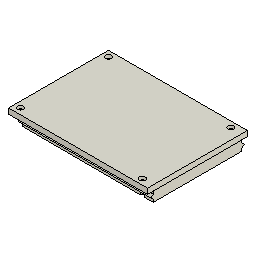
Crashsense Mark-1 LID v10 (Autodesk Fusion 360 design; units mm, degrees)
Autodesk Fusion 360 part; units mm, degrees
note: some values were not read from the file. Chosen so that the rebuilt part matches the saved one: which bodies a step acts on; which face or edge a step refers to. Set by a fixed rule: which sketch regions a step uses.
sketch "Sketch1" plane through (0, 0, 0) normal (0, 0, 1) x (1, 0, 0)
  line L0 (64.0125, -46.025) -> (-64.0125, -46.025)
  line L1 (-64.0125, -46.025) -> (-64.0125, 46.025)
  line L2 (-64.0125, 46.025) -> (64.0125, 46.025)
  line L3 (64.0125, 46.025) -> (64.0125, -46.025)
  line L4 (64.0125, -46.025) -> (-64.0125, 46.025) construction
  line L5 (-64.0125, -46.025) -> (64.0125, 46.025) construction
  line L6 (54.0125, -36.025) -> (-54.0125, -36.025)
  line L7 (-54.0125, -36.025) -> (-54.0125, 36.025)
  line L8 (-54.0125, 36.025) -> (54.0125, 36.025)
  line L9 (54.0125, 36.025) -> (54.0125, -36.025)
  line L10 (54.0125, -36.025) -> (-54.0125, 36.025) construction
  line L11 (-54.0125, -36.025) -> (54.0125, 36.025) construction
  line L12 (54.0125, -36.025) -> (64.0125, -36.025)
  line L13 (54.0125, -36.025) -> (54.0125, -46.025)
  line L14 (54.0125, -46.025) -> (64.0125, -46.025)
  line L15 (54.0125, 36.025) -> (54.0125, 46.025)
  line L16 (54.0125, 36.025) -> (64.0125, 36.025)
  line L17 (-54.0125, 36.025) -> (-64.0125, 36.025)
  line L18 (-54.0125, 36.025) -> (-54.0125, 46.025)
  line L19 (-54.0125, -36.025) -> (-64.0125, -36.025)
  line L20 (-54.0125, -36.025) -> (-54.0125, -46.025)
  line L21 (64.0125, -46.025) -> (64.0125, -36.025)
  line L22 (64.0125, 36.025) -> (64.0125, 46.025)
  line L23 (64.0125, 41.025) -> (-64.0125, 41.025)
  line L24 (-54.0125, 46.025) -> (-64.0125, 46.025)
  line L25 (-59.0125, 46.025) -> (-59.0125, -46.025)
  line L26 (-64.0125, -40.6376) -> (64.0125, -41.025)
  line L27 (64.0125, -41.025) -> (64.0125, -46.025)
  line L28 (-64.0125, -40.6376) -> (-64.0125, -46.025)
  dimension "d1" = 128.025
  dimension "d2" = 92.05
  dimension "d3" = 108.025
  dimension "d4" = 72.05
  constraint horizontal L0
  constraint perpendicular L0 L1
  constraint parallel L0 L2
  constraint parallel L1 L3
  constraint coincident L4 origin
  constraint coincident L5 origin
  constraint horizontal L6
  constraint perpendicular L6 L7
  constraint parallel L6 L8
  constraint parallel L7 L9
  constraint coincident L10 origin
  constraint coincident L11 origin
  constraint coincident L3 L12.end
  constraint perpendicular L3 L12
  constraint coincident L0 L13.end
  constraint perpendicular L0 L13
  constraint coincident L2 L15.end
  constraint perpendicular L2 L15
  constraint coincident L3 L16.end
  constraint perpendicular L3 L16
  constraint coincident L1 L17.end
  constraint perpendicular L1 L17
  constraint coincident L2 L18.end
  constraint perpendicular L2 L18
  constraint coincident L1 L19.end
  constraint perpendicular L1 L19
  constraint coincident L0 L20.end
  constraint perpendicular L0 L20
  constraint midpoint L22 L23.start
  constraint coincident L1 L23.end
  constraint perpendicular L1 L23
  constraint midpoint L24 L25.start
  constraint coincident L0 L25.end
  constraint perpendicular L0 L25
  constraint coincident L1 L26.start
  constraint midpoint L21 L26.end
  measures "d1" distance of L1.end L2.end
  measures "d2" distance of L0.end L1.end
  measures "d3" distance of L7.end L8.end
  measures "d4" distance of L6.end L7.end
extrude "Extrude1" add sketch "Sketch1" along normal blind 10 makes body 1
extrude "Extrude2" add sketch "Sketch1" against normal blind 4 contours L3 L12 L13 L21 L26 | L6 L13 L20 L26 | L3 L9 L12 L16 | L19 L20 L25 L26 | L3 L15 L16 L22 L23 | L7 L17 L19 L25 | L8 L15 L18 L23 | L17 L18 L23 L25 bodies 1
extrude "Extrude3" cut 1 faces at (-18.0042, -40.7768, -1.3333) along direction (0.003026, 0.999995, 0) blind 0.3 on bodies 1 bodies 1
extrude "Extrude4" cut 1 faces at (-59.0125, 13.7991, -1.3333) along direction (1, 0, 0) blind 0.3 on bodies 1 bodies 1
extrude "Extrude5" cut 1 faces at (23.1042, 41.025, -1.3333) along direction (0, -1, 0) blind 0.3 on bodies 1 bodies 1
extrude "Extrude6" cut 1 faces at (60.6792, 12.0083, -4) along direction (0, 0, 1) blind 0.3 on bodies 1 bodies 1
sketch "Sketch2" plane through (0, 0, -3.7) normal (0, 0, -1) x (1, 0, 0)
  line L0 (-58.7125, -40.725) -> (64.0125, -40.725)
  line L1 (64.0125, -40.725) -> (64.0125, 40.725)
  line L2 (64.0125, 40.725) -> (-58.7125, 40.3536)
  line L3 (-58.7125, 40.3536) -> (-58.7125, -40.725)
  line L4 (54.0125, -36.025) -> (-54.0125, -36.025)
  line L5 (-54.0125, -36.025) -> (-54.0125, 36.025)
  line L6 (-54.0125, 36.025) -> (54.0125, 36.025)
  line L7 (54.0125, 36.025) -> (54.0125, -36.025)
sketch "Sketch3" plane through (0, 0, -3.7) normal (0, 0, -1) x (1, 0, 0)
  line L0 (-58.7125, -40.725) -> (64.0125, -40.725)
  line L1 (64.0125, -40.725) -> (64.0125, 40.725)
  line L2 (64.0125, 40.725) -> (-58.7125, 40.3536)
  line L3 (-58.7125, 40.3536) -> (-58.7125, -40.725)
  line L4 (54.0125, -36.025) -> (-54.0125, -36.025)
  line L5 (-54.0125, -36.025) -> (-54.0125, 36.025)
  line L6 (-54.0125, 36.025) -> (54.0125, 36.025)
  line L7 (54.0125, 36.025) -> (54.0125, -36.025)
  circle A0 centre (-58.7125, 40.3536) radius 1.5
  circle A1 centre (-58.7125, -40.725) radius 1.5
  circle A2 centre (54.0125, 40.6947) radius 1.5
  circle A3 centre (54.0125, -40.725) radius 1.5
  dimension "d17" = 3
  dimension "d18" = 3
  dimension "d19" = 3
  dimension "d20" = 3
  constraint coincident L2.end L3.start
  constraint coincident L0.start L3.end
  constraint coincident L2 A2.centre
  constraint coincident L0 A3.centre
  measures "d17" diameter of A0
  measures "d18" diameter of A1
  measures "d19" diameter of A2
  measures "d20" diameter of A3
extrude "Extrude7" cut sketch "Sketch3" against normal blind 100 contours L0 L3 A1 | L0 L3 A1 | L0 A3 | L0 A3 | L2 L3 A0 | L2 L3 A0 | L2 A2 | L2 A2 bodies 1
sketch "Sketch4" plane through (0, 0, 10) normal (0, 0, 1) x (-1, 0, 0)
  circle A0 centre (-54.0125, 40.6947) radius 1.5
  circle A1 centre (58.7125, 40.3536) radius 1.5
  circle A2 centre (-54.0125, -40.725) radius 1.5
  circle A3 centre (58.7125, -40.725) radius 1.5
  line L0 (-64.0125, -46.025) -> (64.0125, -46.025)
  line L1 (64.0125, -46.025) -> (64.0125, 46.025)
  line L2 (64.0125, 46.025) -> (-64.0125, 46.025)
  line L3 (-64.0125, 46.025) -> (-64.0125, -46.025)
  circle A4 centre (58.7125, -40.725) radius 2.65
  circle A5 centre (58.7125, 40.3536) radius 2.65
  circle A6 centre (-54.0125, -40.725) radius 2.65
  circle A7 centre (-54.0125, 40.6947) radius 2.65
  dimension "d23" = 5.3
  dimension "d24" = 5.3
  dimension "d25" = 5.3
  dimension "d26" = 5.3
  constraint concentric A3 A4
  constraint concentric A1 A5
  constraint concentric A2 A6
  constraint concentric A0 A7
  measures "d23" diameter of A4
  measures "d24" diameter of A5
  measures "d25" diameter of A6
  measures "d26" diameter of A7
extrude "Extrude8" cut sketch "Sketch4" against normal blind 2.8 contours A4 | A5 | A6 | A7 bodies 1
extrude "Extrude9" add 1 faces at (60.6792, 12.0083, -3.7) along direction (0, 0, -1) blind 5 on bodies 1 bodies 1
delete_face "DeleteFace1" 2 faces at (-57.9625, 39.426, -7.0333) (-58.4923, 39.2413, 3.5667) on bodies 1
delete_face "DeleteFace2" 2 faces at (-57.2142, -40.2822, -5.3667) (-58.4923, -38.8699, 3.5667) on bodies 1
sketch "Sketch5" plane through (-58.7125, 0, 0) normal (-1, 0, 0) x (0, -1, 0)
  line L0 (40.3536, 0) -> (-40.725, 0)
  line L1 (-40.725, 0) -> (-40.725, -8.7)
  line L2 (-40.725, -8.7) -> (40.3536, -8.7)
  line L3 (40.3536, -8.7) -> (40.3536, 0)
extrude "Extrude10" add 1 faces at (60.6792, 12.0083, -8.7) along direction (0, 0, -1) blind 0.3 on bodies 1 bodies 1
sketch "Sketch6" plane through (-58.7125, 0, 0) normal (-1, 0, 0) x (0, -1, 0)
sketch "Sketch7" plane through (-58.7125, 0, 0) normal (-1, 0, 0) x (0, -1, 0)
  line L0 (40.3536, 0) -> (-40.725, 0)
  line L1 (-40.725, 0) -> (-40.725, -9)
  line L2 (-40.725, -9) -> (40.3536, -9)
  line L3 (40.3536, -9) -> (40.3536, 0)
  line L4 (-40.725, -9) -> (-40.725, 0)
  line L5 (-40.725, 0) -> (-45.725, 0)
  line L6 (-45.725, 0) -> (-45.725, -9)
  line L7 (-45.725, -9) -> (-40.725, -9)
  line L8 (-40.725, -4.5) -> (-45.725, -4.5)
  line L9 (-40.725, -9) -> (-40.725, -4.5)
  line L10 (-40.725, -4.5) -> (-40.725, 0)
  line L11 (-40.725, -2.25) -> (-43.225, -4.5)
  line L12 (-40.725, -6.75) -> (-43.225, -4.5)
  line L13 (-0.1857, -9) -> (-0.1857, 10)
  line L14 (40.3536, -6.75) -> (42.8536, -4.5)
  line L15 (40.3536, -2.25) -> (42.8536, -4.5)
  line L16 (40.3536, -4.5) -> (40.3536, 0)
  dimension "d33" = 5
  constraint coincident L1.end L2.start
  constraint coincident L0.end L1.start
  constraint perpendicular L1 L5
  constraint perpendicular L5 L6
  constraint midpoint L1 L8.start
  constraint midpoint L6 L8.end
  constraint midpoint L10 L11.start
  constraint midpoint L8 L11.end
  constraint midpoint L9 L12.start
  constraint midpoint L2 L13.start
  constraint perpendicular L2 L13
  constraint symmetric L8.start L13 L16.start
  constraint symmetric L0.end L13 L0.start
  constraint symmetric L11.start L13 L15.start
  constraint symmetric L11.end L13 L14.end
  constraint symmetric L12.start L13 L14.start
  measures "d33" distance of L0.end L5.end
extrude "Extrude11" add sketch "Sketch7" against normal blind 122.725 contours L3 L14 L15 L16 | L1 L4 L8 L10 L11 | L1 L4 L8 L9 L12 bodies 1
extrude "Extrude12" cut sketch "Sketch4" against normal blind 100 contours A0 | A1 | A2 | A3 bodies 1
split "Split1" by plane through (0, 0, 0) normal (0, 0, -1) bodies 1 makes body 2 at (60.6792, 12.0083, -9)
move_body "Move1" bodies 2 to x (1, 0, 0) y (0, 1, 0) z (0, 0, 1) at (0, 0, -10)
extrude "Extrude13" cut 3 faces at (-22.9055, -43.2241, 0) (60.6792, 12.0083, 0) (18.0042, -12.0083, 0) along direction (0, 0, 1) blind 5 on bodies 1 bodies 1
move_body "Move2" bodies 2 to x (1, 0, 0) y (0, 1, 0) z (0, 0, 1) at (0, 0, 15)
